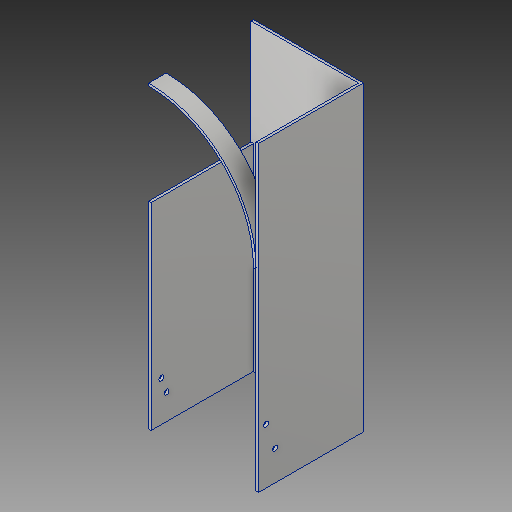
# Autodesk Inventor part: Sorter
Saved by Autodesk Inventor 2019 (Build 230136000, 136)
## iProperties
Created: 2018-11-20
Part Number: Sorter
Material: Aluminum 6061
Document SubType Name: Modeling
Designer: User
Density: 2.7 g/cm^3
Appearance: Aluminum - Flat
Author: User
Autodesk Inventor part; units mm, degrees
ref_plane "YZ Plane" through (0, 0, 0) normal (1, 0, 0) x (0, 1, 0)
ref_plane "XZ Plane" through (0, 0, 0) normal (0, 1, 0) x (-1, 0, 0)
ref_plane "XY Plane" through (0, 0, 0) normal (0, 0, 1) x (1, 0, 0)
sketch "Sketch1" plane through (0, 0, 0) normal (0, 0, 1) x (1, 0, 0)
  line L0 (0, 0) -> (79.9084, 0)
  line L1 (79.9084, 0) -> (79.9084, 219.6084)
  line L2 (79.9084, 219.6084) -> (0, 219.6084)
  line L3 (0, 219.6084) -> (0, 0)
  dimension "d0" = 79.9084
  dimension "d1" = 219.6084
  constraints: 8 end point, 2 parallel, 1 horizontal, 1 perpendicular
  measures "d0" distance of L2.end L1.end
  measures "d1" distance between parallel lines of L2 L0
extrude "Extrusion1" add sketch "Sketch1" along normal blind 76.2
sketch "Sketch2" plane through (0, 0, 0) normal (0, -1, 0) x (1, 0, 0)
  line L0 (79.9084, 0) -> (79.9084, 76.2) projected
  line L1 (0, 0) -> (79.9084, 0) projected
  line L2 (0, 76.2) -> (79.9084, 76.2) projected
  line L3 (78.0542, 1.8542) -> (1.8542, 1.8542)
  line L4 (1.8542, 1.8542) -> (1.8542, 76.2)
  line L5 (1.8542, 76.2) -> (78.0542, 76.2)
  line L6 (78.0542, 76.2) -> (78.0542, 1.8542)
  dimension "d4" = 1.8542
  dimension "d5" = 1.8542
  dimension "d6" = 76.2
  constraints: 8 end point, 2 parallel, 1 horizontal, 1 perpendicular, 1 point on line
  measures "d4" distance from line of L0 L3.start
  measures "d5" distance from line of L1 L3.start
  measures "d6" distance of L4.end L5.end
extrude "Extrusion2" cut sketch "Sketch2" against normal blind 228.6
sketch "Sketch3" plane through (0, 0, 76.2) normal (0, 0, 1) x (1, 0, 0)
  line L0 (1.8542, 0) -> (1.8542, 219.6084) projected
  line L1 (0, 219.6084) -> (1.8542, 219.6084)
  line L2 (1.8542, 219.6084) -> (1.8542, 143.4084)
  line L3 (1.8542, 143.4084) -> (0, 143.4084)
  line L4 (0, 143.4084) -> (0, 219.6084)
  point P0 (0, 0)
  dimension "d9" = 76.2
  constraints: 8 end point, 2 parallel, 1 horizontal, 1 perpendicular, 1 point on line
  measures "d9" distance of L1.end L2.end
extrude "Extrusion3" cut sketch "Sketch3" against normal blind 74.3458
sketch "Sketch9" plane through (0, 0, 76.2) normal (0, 0, 1) x (1, 0, 0)
  line L0 (78.0542, 219.6084) -> (78.0542, 0) projected
  line L1 (0, 143.4084) -> (0, 219.6084) projected
  arc A0 (78.0542, 139.6114) -> (0, 217.6656) centre (0.5141, 140.1255) ccw
  line L2 (0, 217.6656) -> (78.0542, 139.6114) construction
  line L3 (0, 217.6656) -> (110.3853, 217.6656) construction
  line L4 (78.0542, 139.6114) -> (76.2, 139.6114)
  line L5 (0, 217.6656) -> (0, 215.8114)
  arc A1 (76.2, 139.6114) -> (0, 215.8114) centre (0.257, 139.8685) ccw
  point P0 (0, 0)
  dimension "d22" = 45
  dimension "d23" = 1.8542
  dimension "d24" = 1.8542
  constraints: 8 end point, 4 point on circle, 2 centre point, 2 horizontal, 2 point on line, 1 equal length
  measures "d22" angle of L2 L3
  measures "d23" distance of L2.end L4.end
  measures "d24" distance of L2.start L5.end
extrude "Extrusion7" add sketch "Sketch9" against normal blind 12.7
sketch "Sketch10" plane through (0, 0, 0) normal (-1, 0, 0) x (0, 0, 1)
  line L0 (0, 0) -> (76.2, 0) projected
  line L1 (76.2, 143.4084) -> (76.2, 0) projected
  point P0 (64.9986, 18.5674)
  point P1 (68.8594, 29.21)
  dimension "d27" = 18.5674
  dimension "d28" = 11.2014
  dimension "d29" = 7.3406
  dimension "d30" = 29.21
  measures "d27" distance from line of L0 point (64.999, 18.567)
  measures "d28" distance from line of L1 point (64.999, 18.567)
  measures "d29" distance from line of L1 point (68.859, 29.21)
  measures "d30" distance from line of L0 point (68.859, 29.21)
hole "Hole1" at (0, 29.21, 68.8594) at (0, 18.5674, 64.9986) direction (1, 0, 0) diameter 3.7084 depth 1.8542
sketch "Sketch11" plane through (79.9084, 0, 0) normal (1, 0, 0) x (0, 0, -1)
  line L0 (0, 0) -> (-76.2, 0) projected
  line L1 (-76.2, 0) -> (-76.2, 219.6084) projected
  point P0 (-70.7898, 40.1574)
  point P1 (-64.0842, 21.7678)
  dimension "d38" = 40.1574
  dimension "d39" = 5.4102
  dimension "d40" = 12.1158
  dimension "d41" = 21.7678
  measures "d38" distance from line of L0 point (-70.79, 40.157)
  measures "d39" distance from line of L1 point (-70.79, 40.157)
  measures "d40" distance from line of L1 point (-64.084, 21.768)
  measures "d41" distance from line of L0 point (-64.084, 21.768)
hole "Hole2" at (79.9084, 40.1574, 70.7898) at (79.9084, 21.7678, 64.0842) direction (-1, 0, 0) diameter 3.7084 depth 1.8542
body "Solid1"
